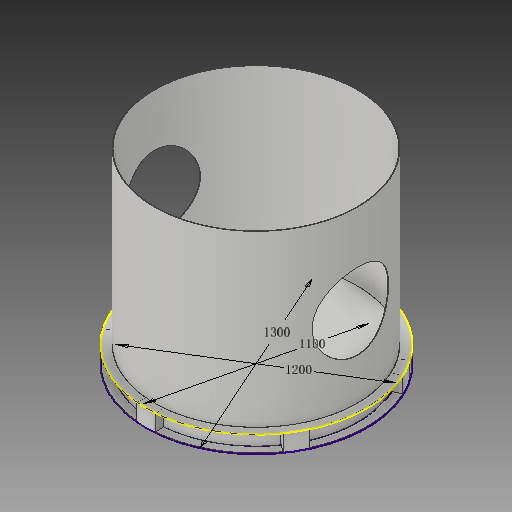
# Autodesk Inventor part: 裙座
Saved by Autodesk Inventor 2018.2 (Build 222227000, 227)
## iProperties
Created: 2018-07-04
Part Number: 裙座
Material: 常规
Document SubType Name: Modeling
Designer: Administrator
Density: 1 g/cm^3
Appearance: 默认
Author: Administrator
Autodesk Inventor part; units mm, degrees
ref_plane "YZ Plane" through (0, 0, 0) normal (1, 0, 0) x (0, 1, 0)
ref_plane "XZ Plane" through (0, 0, 0) normal (0, 1, 0) x (-1, 0, 0)
ref_plane "XY Plane" through (0, 0, 0) normal (0, 0, 1) x (1, 0, 0)
sketch "草图2" plane through (0, 0, 0) normal (0, 1, 0) x (-1, 0, 0)
  circle A0 centre (0, 0) radius 600
  circle A1 centre (0, 0) radius 650
  circle A2 centre (0, 0) radius 550
  dimension "d0" = 1200
  dimension "d10" = 1300
  dimension "d13" = 1100
  constraints: 3 centre point, 3 coincident
  measures "d0" diameter of A0
  measures "d10" diameter of A1
  measures "d13" diameter of A2
surface extrude "拉伸曲面1" sketch "草图2" along normal blind 1100 shown no curves A0
thicken "加厚1" operation new thickness 3.7 both sides no extend neighbours no toward (0.9992617, 0, 0.0384198) faces at (-599.557, 733.3333, -23.0519)
extrude "拉伸2" add sketch "草图2" along normal blind 3.7 contours A1
extrude "拉伸3" add sketch "草图2" along normal blind 3.75 contours A0
ref_plane "工作平面1" through (0, 100, 0) normal (0, -1, 0) x (1, 0, 0)
sketch "草图6" plane through (0, 100, 0) normal (0, -1, 0) x (1, 0, 0)
  circle A0 centre (0, 0) radius 650 projected
extrude "拉伸4" add sketch "草图6" along normal blind 3.75
sketch "草图7" plane through (0, 0, 0) normal (1, 0, 0) x (0, 1, 0)
  line L0 (100, -650) -> (100, 650) projected
  line L1 (0, 650) -> (0, -650) projected
  line L2 (100, -650) -> (0, -650)
  line L3 (0, -650) -> (0, -600)
  line L4 (3.75, 596.3) -> (3.75, -596.3) projected
  line L5 (0, -600) -> (100, -600)
  line L6 (100, -600) -> (1100, -600) projected
  line L7 (-220, 0) -> (1320, 0) projected
  point P0 (0, 0)
  point P1 (96.25, -650)
  point P2 (3.7, -650)
  constraints: 6 end point, 1 collinear, 1 parallel, 1 perpendicular
revolve "旋转1" add sketch "草图7" angle 5 about axis through (0, -10, 0) along (0, 1, 0) and the other way 5 contours L2 L1 L5 L0
pattern_circular "环形阵列1" count 6 over 360 about axis through (0, -10, 0) along (0, 1, 0) of "旋转1"
sketch "草图10" plane through (0, 0, 0) normal (1, 0, 0) x (0, 1, 0)
  circle A0 centre (568.1538, 0) radius 225
  point P0 (0, 0)
  dimension "d26" = 450
  constraints: 1 centre point
  measures "d26" diameter of A0
extrude "拉伸5" cut sketch "草图10" along normal blind 1200 and the other way blind 1200
body "Srf1"
